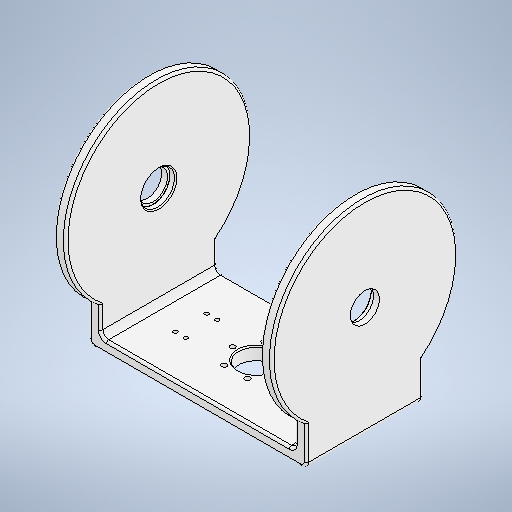
# Autodesk Inventor part: base
Saved by Autodesk Inventor 2025.3 (Build 293356030, 356C)
## iProperties
Created: 2025-08-30
Part Number: base
Material: PLA filament
Document SubType Name: Modeling
Designer: MSI
Density: 1.2 g/cm^3
Appearance: 일반
Mass: 708.037 g
Surface Area: 1330.73 cm^2
Volume: 590.031 cm^3
Author: MSI
Autodesk Inventor part; units mm, degrees
ref_plane "YZ Plane" through (0, 0, 0) normal (1, 0, 0) x (0, 1, 0)
ref_plane "XZ Plane" through (0, 0, 0) normal (0, 1, 0) x (-1, 0, 0)
ref_plane "XY Plane" through (0, 0, 0) normal (0, 0, 1) x (1, 0, 0)
sketch "스케치1" plane through (0, 0, 0) normal (1, 0, 0) x (0, 1, 0)
  circle A0 centre (0, 0) radius 80
  line L0 (0, 50) -> (-96, 50)
  line L1 (-96, 50) -> (-96, -50)
  line L2 (-96, -50) -> (0, -50)
  line L3 (0, -50) -> (0, 50)
  point P0 (-96, 0)
  point P1 (-62.45, -50)
  point P2 (-62.45, 50)
  dimension "d0" = 160
  dimension "d1" = 96
  dimension "d36" = 100
  constraints: 8 end point, 2 coincident, 2 midpoint, 2 parallel, 1 centre point, 1 horizontal, 1 horizontal alignment, 1 perpendicular
  measures "d0" diameter of A0
  measures "d1" distance of L1.end L2.end
  measures "d36" distance of L0.end L1.end
extrude "돌출1" add sketch "스케치1" along normal mid plane 187
sketch "스케치2" plane through (0, 0, 0) normal (0, 0, 1) x (1, 0, 0)
  line L0 (-93.5, 80) -> (93.5, 80) projected
  line L1 (-83.5, 80) -> (83.5, 80)
  line L2 (83.5, 80) -> (83.5, -86)
  line L3 (83.5, -86) -> (-83.5, -86)
  line L4 (-83.5, -86) -> (-83.5, 80)
  line L5 (-93.5, -96) -> (93.5, -96) projected
  line L6 (93.5, -96) -> (93.5, -62.45) projected
  point P0 (0, 0)
  point P1 (0, -86)
  dimension "d4" = 10
  dimension "d5" = 10
  constraints: 8 end point, 2 parallel, 1 horizontal, 1 midpoint, 1 perpendicular, 1 point on line, 1 vertical alignment
  measures "d4" distance between parallel lines of L5 L3
  measures "d5" distance between parallel lines of L6 L2
extrude "돌출2" cut sketch "스케치2" along normal through all both and the other way through all
sketch "스케치3" plane through (-83.5, -86, -50) normal (0, 1, 0) x (1, 0, 0)
  point P0 (83.5, -50)
  point P1 (83.5, -50)
  constraints: 1 coincident
hole "구멍1" at (0, -86, 0) direction (0, -1, 0) diameter 30 end through all
sketch "스케치4" plane through (-83.5, 0, 0) normal (1, 0, 0) x (0, 0, -1)
  arc A0 (50, -62.45) -> (-50, -62.45) centre (0, 0) ccw projected
  point P0 (-80, 0)
  constraints: 1 coincident
hole "구멍2" at (-83.5, 0, 0) direction (-1, 0, 0) diameter 25 end through all counterbore diameter 29 counterbore depth 5
mirror "미러1" about plane through (0, 0, 0) normal (1, 0, 0) of "구멍2"
fillet "모깎기1" radius 5 2 edges at (-83.5, -86, 0) (83.5, -86, 0)
fillet "모깎기2" radius 5 2 edges at (93.5, -96, 0) (-93.5, -96, 0)
fillet "모깎기3" radius 2 24 edges at (-83.5, 80, 0) (-83.5, -71.725, -50) (-82.0355, -84.5355, -50) (0, -86, -50) (82.0355, -84.5355, -50) (83.5, -71.725, -50) (83.5, 80, 0) (83.5, -71.725, 50) (82.0355, -84.5355, 50) (0, -86, 50) (-82.0355, -84.5355, 50) (-83.5, -71.725, 50) (-93.5, 80, 0) (-93.5, -76.725, -50) (-92.0355, -94.5355, -50) (0, -96, -50) (92.0355, -94.5355, -50) (93.5, -76.725, -50) (93.5, 80, 0) (93.5, -76.725, 50) (92.0355, -94.5355, 50) (0, -96, 50) (-92.0355, -94.5355, 50) (-93.5, -76.725, 50)
sketch "스케치8" plane through (-88.5, -96, 48) normal (0, -1, 0) x (1, 0, 0)
  circle A0 centre (88.5, -48) radius 15 projected
  line L0 (62.5192, -48) -> (75.5096, -25.5)
  line L1 (75.5096, -25.5) -> (101.4904, -25.5)
  line L2 (101.4904, -25.5) -> (114.4808, -48)
  line L3 (114.4808, -48) -> (101.4904, -70.5)
  line L4 (101.4904, -70.5) -> (75.5096, -70.5)
  line L5 (75.5096, -70.5) -> (62.5192, -48)
  point P0 (88.5, -48)
  dimension "d65" = 45
  constraints: 12 end point, 1 coincident, 1 horizontal alignment, 13 other
  measures "d65" distance between parallel lines of L4 L1
extrude "돌출3" add sketch "스케치8" along normal blind 1
sketch "스케치5" plane through (-78.5, -86, -48) normal (0, 1, 0) x (1, 0, 0)
  line L0 (78.5, -48) -> (58.5, -48) construction
  dimension "d25" = 20
  constraints: 2 end point, 1 horizontal
  measures "d25" distance of L0.start L0.end
hole "구멍3" at (-20, -86, 0) direction (0, -1, 0) diameter 4.5 end through all clearance for "Socket Head Cap Screw ISO 4762" size "M4" standard "ISO"
pattern_circular "원형 패턴1" count 6 over 360 about axis through (0, -388.564, 0) along (0, 1, 0) of "구멍3"
sketch "스케치6" plane through (-78.5, -96, -48) normal (0, 1, 0) x (1, 0, 0)
  line L0 (19.721, -31.5) -> (34.721, -31.5)
  line L1 (34.721, -31.5) -> (34.721, -64.5)
  line L2 (34.721, -64.5) -> (19.721, -64.5)
  line L3 (19.721, -64.5) -> (19.721, -31.5)
  line L4 (19.721, -31.5) -> (34.721, -64.5) construction
  line L5 (34.721, -31.5) -> (19.721, -64.5) construction
  circle A0 centre (78.5, -48) radius 15 projected
  line L6 (78.5, -33) -> (78.5, -63) construction
  line L7 (137.279, -31.5) -> (122.279, -31.5)
  line L8 (122.279, -31.5) -> (122.279, -64.5)
  line L9 (122.279, -64.5) -> (137.279, -64.5)
  line L10 (137.279, -64.5) -> (137.279, -31.5)
  line L11 (137.279, -31.5) -> (122.279, -64.5) construction
  line L12 (122.279, -31.5) -> (137.279, -64.5) construction
  line L13 (31.721, -61.5) -> (31.721, -34.5)
  line L14 (31.721, -34.5) -> (22.721, -34.5)
  line L15 (22.721, -34.5) -> (22.721, -61.5)
  line L16 (22.721, -61.5) -> (31.721, -61.5)
  line L17 (134.279, -61.5) -> (125.279, -61.5)
  line L18 (125.279, -61.5) -> (125.279, -34.5)
  line L19 (125.279, -34.5) -> (134.279, -34.5)
  line L20 (134.279, -34.5) -> (134.279, -61.5)
  point P0 (27.221, -48)
  point P1 (78.5, -48)
  point P2 (129.779, -48)
  dimension "d37" = 43.779
  dimension "d38" = 15
  dimension "d39" = 33
  dimension "d47" = 3
  dimension "d48" = 3
  constraints: 42 end point, 5 symmetric about line, 4 parallel, 3 midpoint, 2 perpendicular, 2 point on circle, 1 coincident, 1 horizontal, 1 horizontal alignment, 1 vertical, 6 other
  measures "d37" distance from line of point (78.5, -48) L1
  measures "d38" distance of L1.end L2.end
  measures "d39" distance of L2.end L0.start
  measures "d47" distance between parallel lines of L1 L13
  measures "d48" distance between parallel lines of L9 L17
hole "구멍4" at (-55.779, -96, 13.5) at (-46.779, -96, 13.5) at (-46.779, -96, -13.5) at (-55.779, -96, -13.5) at (55.779, -96, 13.5) at (46.779, -96, 13.5) at (46.779, -96, -13.5) at (55.779, -96, -13.5) direction (0, 1, 0) diameter 3.4 end through all counterbore diameter 6.5 counterbore depth 3.3 clearance for "Socket Head Cap Screw ISO 4762" size "M3" standard "ISO"
fillet "모깎기5" radius 3 6 edges at (12.9904, -96.5, 22.5) (25.9808, -96.5, 0) (12.9904, -96.5, -22.5) (-12.9904, -96.5, 22.5) (-25.9808, -96.5, 0) (-12.9904, -96.5, -22.5)
fillet "모깎기4" radius 0.1 2 edges at (-88.5, 0, 14.5) (88.5, 0, 14.5)
chamfer "모따기1" distance 1 angle 45 3 edges at (-83.5, 0, 14.5) (83.5, 0, 14.5) (0, -86, -15)
equation "\"d5\" = d4"
equation "\"d48\" = d47"
